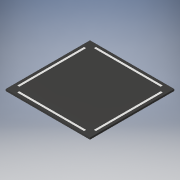
# Autodesk Inventor part: intersection_1
Saved by Autodesk Inventor 2019 (Build 230136000, 136)
## iProperties
Created: 2020-04-29
Part Number: intersection_1
Material: Generic
Document SubType Name: Modeling
Designer: infinity
Density: 1 g/cm^3
Appearance: Smooth - Black
Author: infinity
Autodesk Inventor part; units mm, degrees
ref_plane "YZ Plane" through (0, 0, 0) normal (1, 0, 0) x (0, 1, 0)
ref_plane "XZ Plane" through (0, 0, 0) normal (0, 1, 0) x (-1, 0, 0)
ref_plane "XY Plane" through (0, 0, 0) normal (0, 0, 1) x (1, 0, 0)
sketch "Sketch1" plane through (0, 0, 0) normal (0, 1, 0) x (-1, 0, 0)
  line L0 (0, 0) -> (1219.2, 0)
  line L1 (1219.2, 0) -> (1219.2, -1219.2)
  line L2 (1219.2, -1219.2) -> (0, -1219.2)
  line L3 (0, -1219.2) -> (0, 0)
  dimension "d0" = 1219.2
  dimension "d1" = 1219.2
  constraints: 8 end point, 2 parallel, 1 horizontal, 1 perpendicular
  measures "d0" distance of L0.end L1.end
  measures "d1" distance of L1.end L2.end
extrude "Extrusion1" add sketch "Sketch1" along normal blind 25.4
sketch "Sketch2" plane through (0, 25.4, 0) normal (0, 1, 0) x (1, 0, 0)
  line L0 (-1219.2, 1219.2) -> (-1219.2, 0) projected
  line L1 (0, 1219.2) -> (-1219.2, 1219.2) projected
  line L2 (-1183.0394, 122.6032) -> (-1148.7962, 122.6032)
  line L3 (-1148.7962, 122.6032) -> (-1148.7962, 1096.5968)
  line L4 (-1148.7962, 1096.5968) -> (-1183.0394, 1096.5968)
  line L5 (-1183.0394, 1096.5968) -> (-1183.0394, 122.6032)
  line L6 (-122.6032, 36.1606) -> (-122.6032, 70.4038)
  line L7 (-122.6032, 70.4038) -> (-1096.5968, 70.4038)
  line L8 (-1096.5968, 70.4038) -> (-1096.5968, 36.1606)
  line L9 (-1096.5968, 36.1606) -> (-122.6032, 36.1606)
  line L10 (-36.1606, 1096.5968) -> (-70.4038, 1096.5968)
  line L11 (-70.4038, 1096.5968) -> (-70.4038, 122.6032)
  line L12 (-70.4038, 122.6032) -> (-36.1606, 122.6032)
  line L13 (-36.1606, 122.6032) -> (-36.1606, 1096.5968)
  line L14 (-1096.5968, 1183.0394) -> (-1096.5968, 1148.7962)
  line L15 (-1096.5968, 1148.7962) -> (-122.6032, 1148.7962)
  line L16 (-122.6032, 1148.7962) -> (-122.6032, 1183.0394)
  line L17 (-122.6032, 1183.0394) -> (-1096.5968, 1183.0394)
  point P0 (0, 0)
  point P1 (-609.6, 609.6)
  dimension "d4" = 609.6
  dimension "d5" = 609.6
  dimension "d8" = 360
  constraints: 32 end point, 2 parallel, 1 horizontal, 1 perpendicular, 33 other
  measures "d4" distance from line of point (-609.6, 609.6) L0
  measures "d5" distance from line of point (-609.6, 609.6) L1
extrude "Extrusion2" add sketch "Sketch2" along normal blind 0.254
equation "\"d1\" = d0"
equation "\"d5\" = d4"
body "Solid1"
